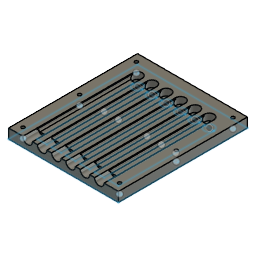
Drosophilla Tracker Stack (Autodesk Fusion 360 design; units mm, degrees)
part number: 2026-08-18-21-22-30-873
Autodesk Fusion 360 part; units mm, degrees
sketch "Sketch1" plane through (0, 0, 0) normal (0, 1, 0) x (1, 0, 0)
  line L0 (0, 40) -> (-10, 40)
  line L1 (-10, 40) -> (-10, -60)
  line L2 (-10, -60) -> (0, -60)
  line L3 (0, -60) -> (0, 40)
  line L4 (15, 40) -> (5, 40)
  line L5 (15, -60) -> (15, 40)
  line L6 (5, 40) -> (5, -60)
  line L7 (5, -60) -> (15, -60)
  line L8 (30, -60) -> (30, 40)
  line L9 (20, -60) -> (30, -60)
  line L10 (30, 40) -> (20, 40)
  line L11 (20, 40) -> (20, -60)
  line L12 (-25, 40) -> (-25, -60)
  line L13 (-15, -60) -> (-15, 40)
  line L14 (-25, -60) -> (-15, -60)
  line L15 (-15, 40) -> (-25, 40)
  line L16 (-30, -60) -> (-30, 40)
  line L17 (-40, 40) -> (-40, -60)
  line L18 (-40, -60) -> (-30, -60)
  line L19 (-30, 40) -> (-40, 40)
  line L20 (45, -60) -> (45, 40)
  line L21 (45, 40) -> (35, 40)
  line L22 (35, -60) -> (45, -60)
  line L23 (35, 40) -> (35, -60)
  circle A0 centre (-35, 40) radius 5
  circle A1 centre (-20, 40) radius 5
  circle A2 centre (-5, 40) radius 5
  circle A3 centre (10, 40) radius 5
  circle A4 centre (25, 40) radius 5
  circle A5 centre (40, 40) radius 5
  line L24 (-55, 60) -> (60, 60)
  line L25 (60, 60) -> (60, -75)
  line L26 (60, -75) -> (-55, -75)
  line L27 (-55, -75) -> (-55, 60)
  circle A6 centre (-48.007, 51.7909) radius 1.7
  circle A7 centre (53.007, 51.7909) radius 1.7
  circle A8 centre (-48.007, -7.5) radius 1.7
  circle A9 centre (53.007, -7.5) radius 1.7
  circle A10 centre (-48.007, -66.7909) radius 1.7
  circle A11 centre (53.007, -66.7909) radius 1.7
  point P0 (15, 0)
  point P1 (30, 0)
  point P2 (-15, 0)
  point P3 (-30, 0)
  point P4 (45, 0)
  dimension "d8" = 100
  dimension "d9" = 10
  dimension "d10" = 100
  dimension "d13" = 10
  dimension "d14" = 10
  dimension "d15" = 10
  dimension "d16" = 10
  dimension "d17" = 10
  dimension "d18" = 10
  dimension "d20" = 3.4
  dimension "d21" = 3.4
  dimension "d22" = 3.4
  dimension "d23" = 3.4
  dimension "d24" = 3.4
  dimension "d25" = 3.4
  dimension "d68" = 135
  dimension "d69" = 115
  dimension "d70" = 59.2909
  dimension "d71" = 59.2909
  dimension "d72" = 101.0141
  dimension "d73" = 59.2909
  dimension "d74" = 59.2909
  constraint horizontal L0
  constraint vertical L1
  constraint horizontal L2
  constraint vertical L3
  constraint horizontal L4
  constraint vertical L6
  constraint horizontal L7
  constraint vertical L5
  constraint horizontal L10
  constraint vertical L11
  constraint horizontal L9
  constraint vertical L8
  constraint horizontal L15
  constraint vertical L12
  constraint horizontal L14
  constraint vertical L13
  constraint horizontal L19
  constraint vertical L17
  constraint horizontal L18
  constraint vertical L16
  constraint horizontal L21
  constraint vertical L23
  constraint horizontal L22
  constraint vertical L20
  constraint midpoint L19 A0.centre
  constraint midpoint L15 A1.centre
  constraint midpoint L0 A2.centre
  constraint midpoint L4 A3.centre
  constraint midpoint L10 A4.centre
  constraint midpoint L21 A5.centre
  constraint horizontal L24
  constraint vertical L25
  constraint horizontal L26
  constraint vertical L27
  measures "d8" distance of L13.end L13.start
  measures "d9" distance of L16.end L17.start
  measures "d10" distance of L16.start L16.end
  measures "d13" diameter of A0
  measures "d14" diameter of A1
  measures "d15" diameter of A2
  measures "d16" diameter of A3
  measures "d17" diameter of A4
  measures "d18" diameter of A5
  measures "d20" diameter of A6
  measures "d21" diameter of A7
  measures "d22" diameter of A8
  measures "d23" diameter of A9
  measures "d24" diameter of A10
  measures "d25" diameter of A11
  measures "d68" distance of L24.end L25.end
  measures "d69" distance of L25.end L26.end
  measures "d70" distance of A8.centre A10.centre
  measures "d71" distance of A6.centre A8.centre
  measures "d72" distance of A6.centre A7.centre
  measures "d73" distance of A7.centre A9.centre
  measures "d74" distance of A9.centre A11.centre
extrude "Extrude11" add sketch "Sketch1" along normal blind 10
extrude "Extrude12" add sketch "Sketch1" along normal blind 7 contours L1 L2 L3 A2 | L5 L6 L7 A3 | L8 L9 L11 A4 | L12 L13 L14 A1 | L16 L17 L18 A0 | L20 L22 L23 A5
extrude "Extrude13" add sketch "Sketch1" along normal blind 3 contours L0 A2 | L0 A2 | L4 A3 | L4 A3 | L10 A4 | L10 A4 | L15 A1 | L15 A1 | L19 A0 | L19 A0 | L21 A5 | L21 A5
hole "Hole7" at (-35.0051, 9.8257, 75) direction (0, 0, -1) diameter 10 depth 16 tip angle 180
hole "Hole8" at (-19.7712, 9.9752, 75) direction (0, 0, -1) diameter 10 depth 16 tip angle 180
hole "Hole9" at (-4.9347, 9.9742, 75) direction (0, 0, -1) diameter 10 depth 16 tip angle 180
hole "Hole10" at (9.9632, 9.9367, 75) direction (0, 0, -1) diameter 10 depth 16 tip angle 180
hole "Hole11" at (24.9361, 9.9742, 75) direction (0, 0, -1) diameter 10 depth 16 tip angle 180
hole "Hole12" at (39.9841, 9.9742, 75) direction (0, 0, -1) diameter 10 depth 16 tip angle 180
fillet "Fillet5" radius 2 tangency weight 0.6 12 edges at (-15, 7, 10) (-30, 7, 10) (0, 7, 10) (15, 7, 10) (30, 7, 10) (45, 7, 10) (35, 7, 10) (20, 7, 10) (5, 7, 10) (-10, 7, 10) (-25, 7, 10) (-40, 7, 10)
sketch "Sketch3" plane through (0, 0, 75) normal (0, 0, 1) x (1, 0, 0)
  arc A0 (34.9841, 10) -> (44.984, 10) centre (39.9841, 9.9742) ccw
  line L0 (34.9841, 10) -> (29.936, 10)
  arc A1 (19.9362, 10) -> (29.936, 10) centre (24.9361, 9.9742) ccw
  line L1 (19.9362, 10) -> (14.9628, 10)
  arc A2 (4.9636, 10) -> (14.9628, 10) centre (9.9632, 9.9367) ccw
  line L2 (4.9636, 10) -> (0.0652, 10)
  arc A3 (-9.9346, 10) -> (0.0652, 10) centre (-4.9347, 9.9742) ccw
  line L3 (-9.9346, 10) -> (-14.7713, 10)
  arc A4 (-24.7712, 10) -> (-14.7713, 10) centre (-19.7712, 9.9752) ccw
  line L4 (-24.7712, 10) -> (-30.0081, 10)
  arc A5 (-40.002, 10) -> (-30.0081, 10) centre (-35.0051, 9.8257) ccw
  line L5 (-40.002, 10) -> (-55, 10)
  line L6 (-55, 10) -> (-55, 0)
  line L7 (-55, 0) -> (60, 0)
  line L8 (60, 0) -> (60, 10)
  line L9 (60, 10) -> (44.984, 10)
